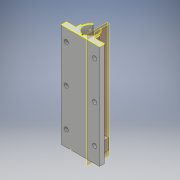
# Autodesk Inventor part: lanceur
Saved by Autodesk Inventor 2017 (Build 210142000, 142)
## iProperties
Part Number: lanceur
Material: Générique
Document SubType Name: Modeling
Designer: Thomas
Density: 1 g/cm^3
Appearance: Par défaut
Author: Thomas
Autodesk Inventor part; units mm, degrees
ref_plane "YZ Plane" through (0, 0, 0) normal (1, 0, 0) x (0, 1, 0)
ref_plane "XZ Plane" through (0, 0, 0) normal (0, 1, 0) x (-1, 0, 0)
ref_plane "XY Plane" through (0, 0, 0) normal (0, 0, 1) x (1, 0, 0)
sketch "Esquisse1" plane through (0, 0, 0) normal (0, 0, 1) x (1, 0, 0)
  line L0 (0, 0) -> (20, 0)
  line L1 (20, 0) -> (20, 20)
  line L2 (20, 20) -> (0, 20)
  line L3 (0, 20) -> (0, 0)
  circle A0 centre (10, 10) radius 2.15
  dimension "d0" = 20
  dimension "d1" = 20
  dimension "d2" = 4.3
  constraints: 8 end point, 2 parallel, 1 centre point, 1 horizontal, 1 perpendicular
  measures "d0" distance of L1.end L2.end
  measures "d1" distance of L0.end L1.end
  measures "d2" diameter of A0
extrude "Extrusion1" add sketch "Esquisse1" along normal blind 4
sketch "Esquisse2" plane through (0, 0, 4) normal (0, 0, 1) x (1, 0, 0)
  circle A0 centre (10, 10) radius 2.15 projected
  line L0 (0, 20) -> (0, 0) projected
  circle A1 centre (10, 10) radius 2.15 projected
  line L1 (0, 0) -> (20, 0) projected
  line L2 (20, 0) -> (20, 20) projected
  line L3 (20, 20) -> (0, 20) projected
  line L4 (0, 20) -> (0, 0) projected
  line L5 (13.4897, 12.0384) -> (13.5102, 7.997)
  line L6 (13.5102, 7.997) -> (10.0204, 5.9586)
  line L7 (10.0204, 5.9586) -> (6.5103, 7.9616)
  line L8 (6.5103, 7.9616) -> (6.4898, 12.003)
  line L9 (6.4898, 12.003) -> (6.4898, 20)
  line L10 (20, 20) -> (0, 20) projected
  line L11 (13.4897, 12.0384) -> (13.4897, 20)
  line L12 (6.4898, 20) -> (0, 20)
  line L13 (0, 0) -> (20, 0) projected
  line L14 (0, 0) -> (0, 20)
  line L15 (0, 0) -> (20, 0)
  line L16 (20, 0) -> (20, 20)
  line L17 (20, 20) -> (13.4897, 20)
  dimension "d5" = 7
  dimension "d6" = 0.29
  constraints: 22 end point, 4 collinear, 3 perpendicular, 2 point on line, 1 coincident, 8 other
  measures "d5" distance between parallel lines of L5 L8
  measures "d6" angle of L0 L8
extrude "Extrusion2" add sketch "Esquisse2" along normal blind 3.2 contours L3 L9 L8 L7 L6 L5 L11 L2 L1 L0
sketch "Esquisse3" plane through (0, 0, 7.2) normal (0, 0, 1) x (1, 0, 0)
  line L0 (6.4898, 20) -> (0, 20) projected
  line L1 (0, 20) -> (20, 20)
  line L2 (20, 20) -> (20, 0)
  line L3 (20, 0) -> (0, 0)
  line L4 (0, 0) -> (0, 20)
  circle A0 centre (10, 10) radius 2.15 projected
  circle A1 centre (10, 10) radius 2.15
  point P0 (0, 0)
  constraints: 8 end point, 2 parallel, 1 centre point, 1 coincident, 1 concentric, 1 horizontal, 1 perpendicular
extrude "Extrusion4" add sketch "Esquisse3" along normal blind 4
sketch "Esquisse4" plane through (0, 0, 11.2) normal (0, 0, 1) x (1, 0, 0)
  line L0 (0, 20) -> (0, 0) projected
  line L1 (0, 10) -> (0, 0)
  line L2 (0, 0) -> (20, 0)
  line L3 (20, 0) -> (20, 10)
  line L4 (20, 0) -> (20, 20) projected
  line L5 (10, 10) -> (2.5, 10) construction
  line L6 (2.5, 10) -> (17.5, 10) construction
  arc A0 (2.5, 10) -> (17.5, 10) centre (10, 10) ccw
  arc A1 (17.5, 10) -> (2.5, 10) centre (10, 10) ccw
  line L7 (0, 10) -> (0, 20)
  line L8 (20, 20) -> (0, 20) projected
  line L9 (0, 20) -> (20, 20)
  line L10 (20, 20) -> (20, 10)
  line L11 (0, 10) -> (1.5, 10)
  line L12 (18.5, 10) -> (20, 10)
  arc A2 (18.5, 10) -> (1.5, 10) centre (10, 10) ccw
  dimension "d15" = 7.5
  dimension "d16" = 1
  constraints: 20 end point, 6 point on circle, 3 centre point, 3 perpendicular, 2 collinear, 2 horizontal, 2 midpoint, 1 concentric, 1 point on line, 1 vertical
  measures "d15" radius of A0
  measures "d16" radial gap between concentric circles of A1 A2
extrude "Extrusion5" add sketch "Esquisse4" along normal blind 20 contours L11 A2 L12 L3 L2 L0
sketch "Esquisse5" plane through (0, 0, 31.2) normal (0, 0, 1) x (1, 0, 0)
  circle A0 centre (10, 10) radius 7.5 projected
  line L0 (0, 0) -> (20, 0) projected
  line L1 (20, 0) -> (20, 10) projected
  line L2 (20, 10) -> (18.5, 10) projected
  arc A1 (18.5, 10) -> (1.5, 10) centre (10, 10) ccw projected
  line L3 (1.5, 10) -> (0, 10) projected
  line L4 (0, 10) -> (0, 0) projected
  arc A2 (18.5, 10) -> (1.5, 10) centre (10, 10) ccw projected
  line L5 (6.0494, 17.5262) -> (6.0494, 16.3752)
  line L6 (13.9506, 16.3752) -> (13.9506, 17.5262)
  arc A3 (18.5, 10) -> (1.5, 10) centre (10, 10) ccw projected
  circle A4 centre (10, 10) radius 7.5 projected
  constraints: 5 point on circle, 4 end point, 1 parallel, 1 vertical
extrude "Extrusion6" add sketch "Esquisse5" along normal blind 78.5 contours A0 L6 A1 L2 L1 L0 L4 L3 L5
sketch "Esquisse6" plane through (0, 0, 109.7) normal (0, 0, 1) x (1, 0, 0)
  arc A0 (6.0494, 16.3752) -> (13.9506, 16.3752) centre (10, 10) ccw projected
  line L0 (0, 0) -> (20, 0) projected
  line L1 (11, 0.567) -> (11, 2.567)
  line L2 (9, 0.567) -> (9, 2.567)
  arc A1 (9, 2.567) -> (11, 2.567) centre (10, 10) ccw
  line L3 (9, 0.567) -> (11, 0.567)
  dimension "d23" = 2
  dimension "d24" = 2
  constraints: 6 end point, 4 point on circle, 1 centre point, 1 horizontal
  measures "d23" distance from line of L3 L2.end
  measures "d24" distance between parallel lines of L1 L2
extrude "Extrusion7" cut sketch "Esquisse6" against normal blind 90
sketch "Esquisse7" plane through (0, 0, 0) normal (-1, 0, 0) x (0, 0, 1)
  point P0 (0, 0)
sketch "Esquisse8" plane through (0, 0, 0) normal (-1, 0, 0) x (0, 0, 1)
  line L0 (109.7, 0) -> (109.7, 10) projected
  line L1 (0, 0) -> (109.7, 0)
  line L2 (109.7, 0) -> (109.7, 5)
  line L3 (109.7, 5) -> (0, 5)
  line L4 (0, 5) -> (0, 0)
  constraints: 8 end point, 2 parallel, 1 horizontal, 1 midpoint, 1 perpendicular
extrude "Extrusion8" add sketch "Esquisse8" along normal blind 10
sketch "Esquisse9" plane through (20, 0, 0) normal (1, 0, 0) x (0, 0, -1)
  line L0 (-109.7, 0) -> (-109.7, 10) projected
  line L1 (0, 0) -> (-109.7, 0)
  line L2 (-109.7, 0) -> (-109.7, 5)
  line L3 (-109.7, 5) -> (0, 5)
  line L4 (0, 5) -> (0, 0)
  constraints: 8 end point, 2 parallel, 1 horizontal, 1 midpoint, 1 perpendicular
extrude "Extrusion9" add sketch "Esquisse9" along normal blind 10
sketch "Esquisse10" plane through (20, 5, 109.7) normal (0, 1, 0) x (1, 0, 0)
  line L0 (10.0235, 93.2538) -> (5.0235, 93.2538) construction
  line L1 (0, 98.5) -> (0, 0) construction
  line L2 (5.0235, 93.2538) -> (5.0235, 8.1061) construction
  circle A0 centre (5.0235, 93.2538) radius 2.15
  circle A1 centre (5.0235, 53.2538) radius 2.15
  circle A2 centre (5.0235, 13.2538) radius 2.15
  circle A3 centre (-24.9765, 93.2538) radius 2.15
  circle A4 centre (-24.9765, 53.2538) radius 2.15
  circle A5 centre (-24.9765, 13.2538) radius 2.15
  point P0 (-20, 109.7)
  dimension "d31" = 5
  dimension "d32" = 4.3
  dimension "d35" = 40
  dimension "d38" = 30
  constraints: 6 centre point, 4 end point, 2 perpendicular, 1 coincident, 1 horizontal, 1 vertical, 10 other
  measures "d31" distance of L0.start L0.end
  measures "d32" diameter of A0
  measures "d35" distance of A0.centre A1.centre
  measures "d38" distance of A0.centre A3.centre
extrude "Extrusion10" cut sketch "Esquisse10" against normal blind 10
sketch "Esquisse11" plane through (0, 0, 109.7) normal (0, 0, 1) x (1, 0, 0)
  line L0 (9, 0.567) -> (9, 2.567) projected
  arc A0 (6.0494, 16.3752) -> (9, 2.567) centre (10, 10) ccw projected
  line L1 (6.0494, 16.3752) -> (6.0494, 17.5262) projected
  arc A1 (6.0494, 17.5262) -> (1.5, 10) centre (10, 10) ccw projected
  line L2 (1.5, 10) -> (0, 10) projected
  line L3 (0, 10) -> (0, 5) projected
  line L4 (0, 5) -> (-10, 5) projected
  line L5 (-10, 0) -> (-10, 5) projected
  line L6 (30, 0) -> (-10, 0) projected
  line L7 (30, 5) -> (30, 0) projected
  line L8 (20, 5) -> (30, 5) projected
  line L9 (20, 5) -> (20, 10) projected
  line L10 (20, 10) -> (18.5, 10) projected
  arc A2 (18.5, 10) -> (13.9506, 17.5262) centre (10, 10) ccw projected
  line L11 (13.9506, 17.5262) -> (13.9506, 16.3752) projected
  arc A3 (11, 2.567) -> (13.9506, 16.3752) centre (10, 10) ccw projected
  line L12 (11, 2.567) -> (11, 0.567) projected
  line L13 (11, 0.567) -> (9, 0.567) projected
  point P0 (0, 0)
ref_plane "Plan de construction1" through (17.5, 10, 11.2) normal (1, 0, 0) x (0, 1, 0)
ref_plane "Plan de construction2" through (20, 20, 11.2) normal (1, 0, 0) x (0, 0, -1)
